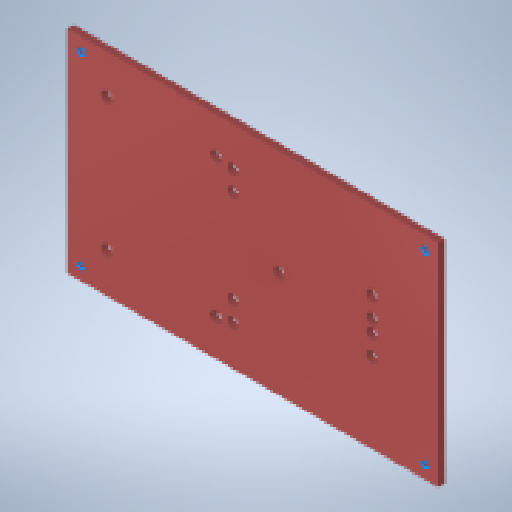
# Autodesk Inventor part: BaseEnsamble
Saved by Autodesk Inventor 2023.1 (Build 271208000, 208)
## iProperties
Created: 2022-11-01
Part Number: BaseEnsamble
Material: MDF Medium Density Fiberboard
Document SubType Name: Modeling
Designer: Daniel Peña
Density: 0.8 g/cm^3
Appearance: Chestnut
Author: Daniel Peña
Autodesk Inventor part; units mm, degrees
ref_plane "YZ Plane" through (0, 0, 0) normal (1, 0, 0) x (0, 1, 0)
ref_plane "XZ Plane" through (0, 0, 0) normal (0, 1, 0) x (-1, 0, 0)
ref_plane "XY Plane" through (0, 0, 0) normal (0, 0, 1) x (1, 0, 0)
sketch "Sketch1" plane through (0, 0, 0) normal (0, 0, 1) x (1, 0, 0)
  line L0 (-200, 20) -> (80, 20)
  line L1 (80, 20) -> (80, -140)
  line L2 (80, -140) -> (-200, -140)
  line L3 (-200, -140) -> (-200, 20)
  point P0 (0, 0)
  dimension "d0" = 280
  dimension "d1" = 160
  dimension "d2" = 80
  dimension "d3" = 140
  constraints: 8 end point, 2 parallel, 1 horizontal, 1 perpendicular
  measures "d0" distance of L1.end L2.end
  measures "d1" distance of L0.end L1.end
  measures "d2" distance from line of point (0, 0) L1
  measures "d3" distance from line of L2 point (0, 0)
extrude "Extrusion1" add sketch "Sketch1" along normal blind 5
sketch "Sketch2" plane through (0, 0, 5) normal (0, 0, 1) x (1, 0, 0)
  circle A0 centre (50.3964, 47.2827) radius 2.5 projected
  point P0 (0, 0)
  point P1 (-87.5, -7.5)
  point P2 (-170, -10)
  point P3 (-170, -110)
  point P4 (-87.5, -112.5)
  point P5 (-75, -109.875)
  point P6 (-75, -94.875)
  point P7 (-75, -24.875)
  point P8 (-75, -9.875)
  point P9 (-39.999, -60)
  point P10 (30.0009, -79.878)
  point P11 (30.0009, -64.878)
  point P12 (30.0008, -54.872)
  point P13 (30.0008, -39.872)
hole "TornillosGripper" at (-87.5, -7.5, 5) at (-170, -10, 5) at (-170, -110, 5) at (-87.5, -112.5, 5) at (-75, -109.875, 5) at (-75, -94.875, 5) at (-75, -24.875, 5) at (-75, -9.875, 5) at (-39.999, -60, 5) at (30.0009, -79.878, 5) at (30.0009, -64.878, 5) at (30.0008, -54.872, 5) at (30.0008, -39.872, 5) direction (0, 0, -1) diameter 8.5 end through all
sketch "Sketch3" plane through (0, 0, 5) normal (0, 0, 1) x (1, 0, 0)
  line L0 (80, 20) -> (-200, 20) projected
  line L1 (-60, 20) -> (-60, -140) construction
  line L2 (-200, -140) -> (80, -140) projected
  line L3 (-200, 20) -> (-200, -140) projected
  line L4 (-200, -60) -> (80, -60) construction
  line L5 (80, -140) -> (80, 20) projected
  point P0 (0, 0)
  point P1 (-190, 10)
  point P2 (-190, -130)
  point P3 (70, -130)
  point P4 (70, 10)
  point P5 (50, 10)
  point P6 (50, -130)
  dimension "d13" = 10
  dimension "d14" = 10
  dimension "d22" = 20
  dimension "d23" = 10
  constraints: 5 symmetric about line, 4 end point, 4 midpoint
  measures "d13" distance from line of L0 point (-190, 10)
  measures "d14" distance from line of point (-190, 10) L3
  measures "d22" distance of point (70, 10) point (50, 10)
  measures "d23" distance from line of L0 point (50, 10)
hole "TornillosBase" at (-190, 10, 5) at (-190, -130, 5) at (70, -130, 5) at (70, 10, 5) at (50, 10, 5) at (50, -130, 5) direction (0, 0, -1) diameter 5 end through all
equation "\"d2\" = 0.5 * d1"
equation "\"d3\" = 0.5 * d0"
body "Solid1"
